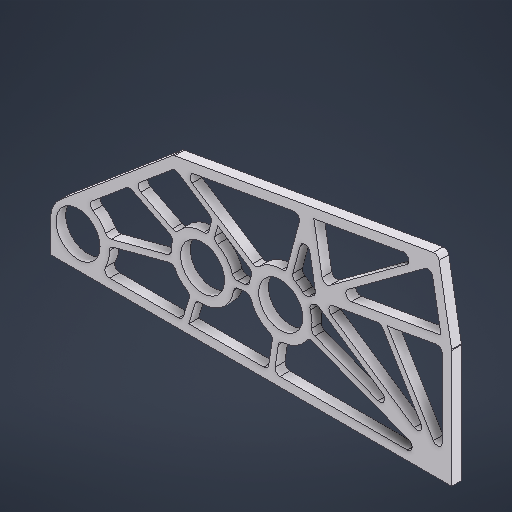
# Autodesk Inventor part: INTAKE_OUTSIDE_PLATE
Saved by Autodesk Inventor 2026.2 (Build 302298010, 298A)
## iProperties
Created: 2026-04-01
Part Number: INTAKE_OUTSIDE_PLATE
Material: Aluminum, 6061-T6
Document SubType Name: Sheet Metal
Designer: 4aida
Density: 2.71 g/cm^3
Appearance: Metal-AL-6061 (Flat)
Sheet Metal Rule: Default
Author: 4aida
Autodesk Inventor part; units mm, degrees
ref_plane "YZ Plane" through (0, 0, 0) normal (1, 0, 0) x (0, 1, 0)
ref_plane "XZ Plane" through (0, 0, 0) normal (0, 1, 0) x (-1, 0, 0)
ref_plane "XY Plane" through (0, 0, 0) normal (0, 0, 1) x (1, 0, 0)
sketch "Sketch1" plane through (0, 0, 0) normal (0, 0, 1) x (1, 0, 0)
  circle A0 centre (0, 0) radius 14.2875
  line L0 (-17.78, -20.5105) -> (242.0644, -20.5105)
  line L1 (-17.78, -20.5105) -> (-17.78, 0)
  line L2 (-11.4288, 13.6203) -> (61.7316, 75.0091)
  line L3 (241.0225, 61.8426) -> (234.4065, 99.3638) construction
  line L4 (234.4065, 99.3638) -> (-12.4495, 55.8365) construction
  line L5 (-12.4495, 55.8365) -> (-5.8335, 18.3153) construction
  circle A1 centre (0, 0) radius 19.05 construction
  circle A2 centre (131.3259, 25.7355) radius 19.05 construction
  line L6 (61.7316, 75.0091) -> (233.3646, 105.2727)
  line L7 (233.3646, 105.2727) -> (242.0644, 55.9338)
  line L8 (242.0644, 55.9338) -> (242.0644, -20.5105)
  line L9 (242.0644, 55.9338) -> (233.3646, 105.2727)
  line L10 (233.3646, 105.2727) -> (141.5413, 89.0817)
  circle A3 centre (131.3259, 25.7355) radius 14.2875
  arc A4 (-11.4288, 13.6203) -> (-17.78, 0) centre (0, 0) ccw
  line L11 (-5.8335, 18.3153) -> (147.6287, 45.3748) construction
  line L12 (147.6287, 45.3748) -> (241.0225, 61.8426) construction
  line L13 (233.3646, 105.2727) -> (242.0644, 55.9338)
  circle A5 centre (80.7113, 21.3995) radius 14.2875
  circle A6 centre (80.7113, 21.3995) radius 40.64 construction
  line L14 (131.3259, 25.7355) -> (80.7113, 21.3995)
  dimension "d0" = 28.575
  dimension "d2" = 20.5105
  dimension "d5" = 38.1
  dimension "d6" = 38.1
  dimension "d8" = 6
  dimension "d18" = 28.575
  dimension "d23" = 38.1
  dimension "d24" = 17.78
  dimension "d25" = 10
  dimension "d26" = 30
  dimension "d31" = 50.1
  dimension "d32" = 114.3
  dimension "d35" = 60.61
  dimension "d80" = 28.575
  dimension "d81" = 50.8
  dimension "d82" = 81.28
  dimension "d83" = 41.91
  dimension "d101" = 83.5
  constraints: 30 end point, 8 perpendicular, 7 centre point, 6 coincident, 3 tangent, 2 point on circle, 2 point on line, 1 collinear, 1 horizontal
  measures "d0" diameter of A0
  measures "d2" distance from line of point (0, 0) L0
  measures "d5" diameter of A1
  measures "d6" diameter of A2
  measures "d8" distance between parallel lines of L6 L4
  measures "d18" diameter of A3
  measures "d23" distance between parallel lines of L4 L11
  measures "d24" radius of A4
  measures "d25" angle of L11 L0
  measures "d26" angle of L2 L11
  measures "d31" distance of L6.end L7.end
  measures "d32" distance from line of L7 A2.centre
  measures "d35" distance from line of L6 A2.centre
  measures "d80" diameter of A5
  measures "d81" distance of L14.start L14.end
  measures "d82" diameter of A6
  measures "d83" distance from line of A5.centre L0
  measures "d101" distance of L14.end point (0, 0)
extrude "Extrusion1" add sketch "Sketch1" along normal blind 6.35
sketch "Sketch2" plane through (0, 0, 6.35) normal (0, 0, 1) x (1, 0, 0)
  line L0 (242.0644, 55.9338) -> (233.3646, 105.2727) projected
  line L1 (233.3646, 105.2727) -> (61.7316, 75.0091) projected
  line L2 (61.7316, 75.0091) -> (-11.4288, 13.6203) projected
  arc A0 (-11.4288, 13.6203) -> (-17.78, 0) centre (0, 0) ccw projected
  line L3 (-17.78, 0) -> (-17.78, -20.5105) projected
  line L4 (-17.78, -20.5105) -> (242.0644, -20.5105) projected
  line L5 (242.0644, -20.5105) -> (242.0644, 55.9338) projected
  circle A1 centre (0, 0) radius 14.2875 projected
  circle A2 centre (131.3259, 25.7355) radius 14.2875 projected
  line L6 (64.3568, 69.3795) -> (228.4977, 98.3219)
  line L7 (228.4977, 98.3219) -> (236.0644, 55.4089)
  line L8 (236.0644, 55.4089) -> (236.0644, -14.5105)
  line L9 (236.0644, -14.5105) -> (14.1784, -14.5105)
  line L10 (5.0808, 19.641) -> (64.3568, 69.3795)
  arc A3 (14.1784, -14.5105) -> (5.0808, 19.641) centre (0, 0) ccw
  circle A4 centre (131.3259, 25.7355) radius 20.2875
  line L11 (154.515, 40.4965) -> (242.0644, 55.9338)
  line L12 (242.0644, 55.9338) -> (233.3646, 105.2727)
  line L13 (233.3646, 105.2727) -> (145.8152, 89.8353)
  line L14 (145.8152, 89.8353) -> (154.515, 40.4965)
  line L15 (154.515, 40.4965) -> (233.3646, 105.2727) construction
  line L16 (242.0644, 55.9338) -> (145.8152, 89.8353) construction
  circle A5 centre (131.3259, 25.7355) radius 31.75 construction
  line L17 (235.1136, 60.8008) -> (159.3819, 47.4472)
  line L18 (159.3819, 47.4472) -> (152.7659, 84.9684)
  line L19 (152.7659, 84.9684) -> (228.4977, 98.3219)
  line L20 (228.4977, 98.3219) -> (235.1136, 60.8008)
  line L21 (235.1136, 60.8008) -> (152.7659, 84.9684) construction
  line L22 (159.3819, 47.4472) -> (228.4977, 98.3219) construction
  line L23 (154.515, 40.4965) -> (236.0644, -14.5105) construction
  line L24 (198.2897, 48.2151) -> (236.0644, -14.5105) construction
  line L25 (154.4832, 38.1054) -> (220.3721, -6.3381)
  line L26 (157.3503, 40.9964) -> (229.6858, -7.7956)
  line L27 (196.1791, 47.843) -> (229.6858, -7.7956)
  line L28 (200.4002, 48.5873) -> (236.0644, -10.6337)
  line L29 (115.504, 38.4339) -> (67.2398, 69.8878)
  line L30 (114.3292, 36.8123) -> (64.3568, 69.3795) construction
  line L31 (113.32, 35.0828) -> (62.7555, 68.0358)
  line L32 (126.2732, 6.0873) -> (123.0978, -14.5105)
  line L33 (128.2348, 5.6849) -> (125.1214, -14.5105) construction
  line L34 (130.2265, 5.4778) -> (127.145, -14.5105)
  line L35 (149.4538, 16.6272) -> (230.4884, -14.5105)
  line L36 (150.2635, 18.4587) -> (236.0644, -14.5105) construction
  line L37 (150.8886, 20.3611) -> (220.3721, -6.3381)
  line L38 (148.4402, 36.6296) -> (154.515, 40.4965) construction
  line L39 (147.2829, 38.2637) -> (154.1391, 42.628)
  line L40 (138.4644, 44.7256) -> (147.6806, 79.2562)
  line L41 (136.5575, 45.3368) -> (146.8571, 83.9265) construction
  line L42 (134.5997, 45.7571) -> (144.6849, 83.5435)
  line L43 (149.4309, 34.8894) -> (154.4832, 38.1054)
  line L44 (154.9393, 46.9598) -> (155.2373, 47.1495)
  line L45 (228.4977, 98.3219) -> (159.3819, 47.4472) construction
  line L46 (163.8185, 48.2295) -> (228.8852, 96.1238)
  line L47 (158.9943, 49.6453) -> (224.0611, 97.5396)
  circle A6 centre (80.7113, 21.3995) radius 14.2875 projected
  circle A7 centre (80.7113, 21.3995) radius 20.2819
  line L48 (80.7113, 21.3995) -> (69.6499, -14.5105) construction
  line L49 (80.7113, 21.3995) -> (89.343, 53.0959) construction
  line L50 (80.7113, 21.3995) -> (34.7188, 44.5102) construction
  line L51 (36.3872, 45.9102) -> (68.9686, 29.5384)
  line L52 (84.0848, 41.3989) -> (87.0305, 52.2157)
  line L53 (71.7427, -14.5105) -> (76.6812, 1.522)
  line L54 (67.5572, -14.5105) -> (72.8584, 2.6996)
  line L55 (60.6897, 18.1602) -> (19.0019, 7.1072)
  line L56 (33.0504, 43.1103) -> (67.1726, 25.9642)
  line L57 (61.7149, 14.2938) -> (20.027, 3.2408)
  line L58 (0, 0) -> (80.7113, 21.3995) construction
  line L59 (80.7113, 21.3995) -> (131.3259, 25.7355) construction
  line L60 (87.9442, 40.3478) -> (90.5513, 49.9212)
  line L61 (100.65, 25.1149) -> (111.0402, 26.005)
  line L62 (111.3816, 22.0196) -> (100.9702, 21.1277)
  point P0 (193.9398, 72.8846)
  point P1 (126.6781, -4.4128)
  point P2 (236.0644, 54.8758)
  point P3 (124.2242, -14.5105)
  point P4 (228.8852, 96.1238)
  point P5 (224.0611, 97.5396)
  point P6 (152.7659, 84.9684)
  point P7 (120.1743, -14.5105)
  point P8 (106.1759, 21.5736)
  point P9 (84.3211, 52.3108)
  point P10 (87.6721, 49.8617)
  point P11 (100.9914, 21.1295)
  point P12 (70.2223, -14.5105)
  point P13 (63.575, 32.2486)
  point P14 (61.779, 28.6745)
  dimension "d41" = 63.5
  dimension "d37" = 6
  dimension "d38" = 6
  dimension "d39" = 6
  dimension "d40" = 88.9
  dimension "d42" = 6
  dimension "d43" = 6
  dimension "d55" = 2
  dimension "d56" = 2
  dimension "d57" = 2
  dimension "d58" = 2
  dimension "d62" = 2
  dimension "d63" = 2
  dimension "d66" = 2
  dimension "d67" = 2
  dimension "d68" = 2
  dimension "d69" = 2
  dimension "d70" = 2
  dimension "d71" = 2
  dimension "d72" = 2
  dimension "d73" = 2
  dimension "d77" = 2
  dimension "d78" = 2
  dimension "d84" = 5.9944
  dimension "d85" = 110.943
  dimension "d86" = 55.4715
  dimension "d87" = 2
  dimension "d91" = 2
  dimension "d93" = 2
  dimension "d94" = 2
  dimension "d95" = 2
  dimension "d96" = 2
  dimension "d97" = 2
  dimension "d98" = 2
  dimension "d99" = 2
  dimension "d102" = 2
  constraints: 113 end point, 26 parallel, 25 point on line, 9 midpoint, 6 point on circle, 2 perpendicular, 1 centre point, 1 coincident, 43 other
  measures "d37" distance between parallel lines of L1 L6
  measures "d38" radial gap between concentric circles of A1 A3
  measures "d40" distance between parallel lines of L0 L14
  measures "d42" distance between parallel lines of L2 L10
  measures "d55" distance between parallel lines of L23 L25
  measures "d56" distance between parallel lines of L23 L26
  measures "d57" distance between parallel lines of L24 L27
  measures "d58" distance between parallel lines of L24 L28
  measures "d62" distance between parallel lines of L29 L30
  measures "d63" distance between parallel lines of L30 L31
  measures "d66" distance from line of point (126.678, -4.413) L32
  measures "d67" distance between parallel lines of L34 L33
  measures "d68" distance between parallel lines of L36 L35
  measures "d69" distance between parallel lines of L37 L36
  measures "d70" distance between parallel lines of L41 L40
  measures "d71" distance between parallel lines of L41 L42
  measures "d72" distance between parallel lines of L38 L39
  measures "d73" distance between parallel lines of L43 L38
  measures "d77" distance between parallel lines of L22 L46
  measures "d78" distance between parallel lines of L22 L47
  measures "d85" distance of A3.start L33.end
  measures "d86" distance of L48.end A3.start
  measures "d87" distance between parallel lines of L50 L51
  measures "d91" distance between parallel lines of L57 L58
  measures "d93" distance between parallel lines of L48 L54
  measures "d94" distance between parallel lines of L53 L48
  measures "d95" distance between parallel lines of L49 L60
  measures "d96" distance between parallel lines of L52 L49
  measures "d97" distance between parallel lines of L61 L59
  measures "d98" distance from line of L59 point (106.176, 21.574)
  measures "d99" distance between parallel lines of L58 L55
  measures "d102" distance between parallel lines of L50 L56
extrude "Cut1" cut sketch "Sketch2" against normal through all contours L8 L28 L11 | L17 L46 L7 | L27 L26 L11 | L42 A4 L29 L6 | L6 L47 L18 | L14 L39 A4 L40 | L9 L34 A4 L35 | L9 L53 A7 L62 A4 L32 | A4 L43 L25 L37 | L31 L52 A7 L51 L10 | A4 L61 A7 L60 L31 | L9 A3 L57 A7 L54 | L56 A7 L55 A3 L10 | A6 | A2
fillet "Fillet1" radius 3.175 36 edges at (62.7555, 68.0358, 3.175) (67.2398, 69.8878, 3.175) (14.1784, -14.5105, 3.175) (19.0019, 7.1072, 3.175) (20.027, 3.2408, 3.175) (5.0808, 19.641, 3.175) (113.32, 35.0828, 3.175) (115.504, 38.4339, 3.175) (134.5997, 45.7571, 3.175) (138.4644, 44.7256, 3.175) (147.2829, 38.2637, 3.175) (149.4309, 34.8894, 3.175) (150.8886, 20.3611, 3.175) (149.4538, 16.6272, 3.175) (130.2265, 5.4778, 3.175) (126.2732, 6.0873, 3.175) (230.4884, -14.5105, 3.175) (220.3721, -6.3381, 3.175) (229.6858, -7.7956, 3.175) (236.0644, -10.6337, 3.175) (154.4832, 38.1054, 3.175) (196.1791, 47.843, 3.175) (157.3503, 40.9964, 3.175) (236.0644, 54.8758, 3.175) (154.1391, 42.628, 3.175) (147.6806, 79.2562, 3.175) (144.6849, 83.5435, 3.175) (163.8185, 48.2295, 3.175) (158.9943, 49.6453, 3.175) (228.8852, 96.1238, 3.175) (224.0611, 97.5396, 3.175) (233.3646, 105.2727, 3.175) (242.0644, 55.9338, 3.175) (61.7316, 75.0091, 3.175) (123.0978, -14.5105, 3.175) (127.145, -14.5105, 3.175)
fillet "Fillet2" radius 3.175 16 edges at (87.0305, 52.2157, 3.175) (87.9442, 40.3478, 3.175) (84.0848, 41.3989, 3.175) (63.575, 32.2486, 3.175) (61.779, 28.6745, 3.175) (33.0504, 43.1103, 3.175) (36.3872, 45.9102, 3.175) (61.7149, 14.2938, 3.175) (60.6897, 18.1602, 3.175) (67.5572, -14.5105, 3.175) (76.6812, 1.522, 3.175) (72.8584, 2.6996, 3.175) (100.9914, 21.1295, 3.175) (111.3816, 22.0196, 3.175) (100.65, 25.1149, 3.175) (111.0402, 26.005, 3.175)
equation "\"d9\" = d8"
equation "\"BendRadius\" = Thickness"
equation "\"BendReliefWidth\" = Thickness"
equation "\"BendReliefDepth\" = 0.5 * Thickness"
equation "\"CornerReliefSize\" = 4 * Thickness"
equation "\"MinimumRemnant\" = 2 * Thickness"
equation "\"TransitionRadius\" = BendRadius"
equation "\"JacobiRadiusSize\" = BendRadius"
equation "\"GapSize\" = Thickness"
equation "\"d22\" = d8"
equation "\"Thickness\" = 3.048"
body "Solid1"
